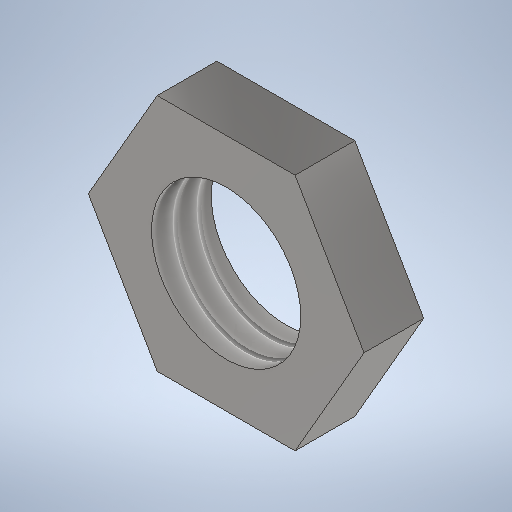
# Autodesk Inventor part: Resistencia_Tuerca
Saved by Autodesk Inventor 2026 (Build 300175050, 175E)
## iProperties
Created: 2025-05-26
Part Number: Resistencia_Tuerca
Material: Acero, suave
Document SubType Name: Modeling
Designer: alex
Density: 7.85 g/cm^3
Appearance: Semipulido
Author: alex
Autodesk Inventor part; units mm, degrees
ref_plane "YZ Plane" through (0, 0, 0) normal (1, 0, 0) x (0, 1, 0)
ref_plane "XZ Plane" through (0, 0, 0) normal (0, 1, 0) x (-1, 0, 0)
ref_plane "XY Plane" through (0, 0, 0) normal (0, 0, 1) x (1, 0, 0)
sketch "Boceto1" plane through (0, 0, 0) normal (0, 0, 1) x (1, 0, 0)
  circle A0 centre (0, 0) radius 2.5
  line L0 (2.3094, 4) -> (4.6188, 0)
  line L1 (4.6188, 0) -> (2.3094, -4)
  line L2 (2.3094, -4) -> (-2.3094, -4)
  line L3 (-2.3094, -4) -> (-4.6188, 0)
  line L4 (-4.6188, 0) -> (-2.3094, 4)
  line L5 (-2.3094, 4) -> (2.3094, 4)
  dimension "d0" = 5
  dimension "d1" = 4
  constraints: 12 end point, 2 coincident, 1 centre point, 13 other
  measures "d0" diameter of A0
  measures "d1" distance from line of L5 point (0, 0)
extrude "Extrusión1" add sketch "Boceto1" along normal mid plane 2
thread "Rosca1" size "M5x0.8" class "6H" standard "ANSI Metric M Profile" full length
